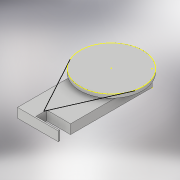
# Autodesk Inventor part: Part2
Saved by Autodesk Inventor 2019 (Build 230136000, 136)
## iProperties
Created: 2020-02-18
Part Number: Part2
Material: Generic
Document SubType Name: Modeling
Designer: Lenovo
Density: 1 g/cm^3
Appearance: Default
Author: Lenovo
Autodesk Inventor part; units mm, degrees
ref_plane "YZ Plane" through (0, 0, 0) normal (1, 0, 0) x (0, 1, 0)
ref_plane "XZ Plane" through (0, 0, 0) normal (0, 1, 0) x (-1, 0, 0)
ref_plane "XY Plane" through (0, 0, 0) normal (0, 0, 1) x (1, 0, 0)
sketch "Sketch1" plane through (0, 0, 0) normal (0, 1, 0) x (-1, 0, 0)
  line L0 (0, 0) -> (13.0401, 0)
  line L1 (13.0401, 0) -> (13.0401, 30.019)
  line L2 (13.0401, 30.019) -> (0, 30.019)
  line L3 (0, 30.019) -> (0, 0)
  constraints: 8 end point, 2 parallel, 1 horizontal, 1 perpendicular
extrude "Extrusion1" add sketch "Sketch1" along normal blind 3
sketch "Sketch2" plane through (0, 3, 0) normal (0, 1, 0) x (1, 0, 0)
  circle A0 centre (-6.6543, -6.3858) radius 0.7285
  point P0 (0, 0)
  constraints: 1 centre point
extrude "Extrusion2" add sketch "Sketch2" along normal blind 1
sketch "Sketch3" plane through (-6.6543, 4, 6.3858) normal (0, 1, 0) x (1, 0, 0)
  point P0 (6.6543, 6.3858)
sketch "Sketch4" plane through (-6.6543, 4, 6.3858) normal (0, 1, 0) x (1, 0, 0)
  circle A0 centre (0, 0) radius 0.7285 projected
  circle A1 centre (0, 0) radius 10.0143
  point P0 (6.6543, 6.3858)
  constraints: 1 centre point, 1 coincident
extrude "Extrusion3" add sketch "Sketch4" along normal blind 1
sketch "Sketch5" plane through (0, 0, 30.019) normal (1, 0, 0) x (0, 0, -1)
  point P0 (30.019, 0)
sketch "Sketch6" plane through (0, 3, 0) normal (0, 1, 0) x (1, 0, 0)
  line L0 (0, -30.019) -> (0, 0) projected
  line L1 (0, -28.1093) -> (-7.3705, -28.1093)
  line L2 (-7.3705, -28.1093) -> (-7.3705, -24.1704)
  line L3 (-7.3705, -24.1704) -> (0, -24.1704)
  line L4 (0, -24.1704) -> (0, -28.1093)
  constraints: 8 end point, 2 parallel, 1 horizontal, 1 perpendicular, 1 point on line
extrude "Extrusion4" add sketch "Sketch6" against normal blind 1
sketch "Sketch7" plane through (0, 3, 0) normal (0, 1, 0) x (1, 0, 0)
  line L0 (0, -30.019) -> (0, 0) projected
  line L1 (0, -26.0801) -> (-7.6092, -26.0801)
  line L2 (-7.6092, -26.0801) -> (-7.6092, -29.5416)
  line L3 (-7.6092, -29.5416) -> (0, -29.5416)
  line L4 (0, -29.5416) -> (0, -26.0801)
  constraints: 8 end point, 2 parallel, 1 horizontal, 1 perpendicular, 1 point on line
extrude "Extrusion5" cut sketch "Sketch7" against normal blind 3
sketch "Sketch8" plane through (-6.6543, 5, 6.3858) normal (0, 1, 0) x (1, 0, 0)
  circle A0 centre (0, 0) radius 10.0143 projected
  line L0 (-6.3858, -23.6333) -> (6.6543, -23.6333) projected
  point P0 (6.6543, 6.3858)
sketch "Sketch9" plane through (-6.6543, 5, 6.3858) normal (0, 1, 0) x (1, 0, 0)
  point P0 (6.6543, 6.3858)
extrude "Extrusion6" add sketch "Sketch8" along normal blind 0.2
sketch "Sketch10" plane through (-6.6543, 5.2, 6.3858) normal (0, 1, 0) x (1, 0, 0)
  circle A0 centre (0, 0) radius 10.0143 projected
  line L0 (-9.1289, -4.117) -> (1.0146, -22.6784)
  line L1 (1.0146, -22.6784) -> (9.9069, -2.4469)
  point P0 (6.6543, 6.3858)
  constraints: 4 end point, 2 other
body "Solid1"
